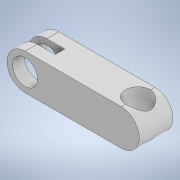
# Autodesk Inventor part: toplegV2
Saved by Autodesk Inventor 2022 (Build 260153000, 153)
## iProperties
Created: 2022-01-24
Part Number: toplegV2
Material: Generic
Document SubType Name: Modeling
Designer: money
Density: 1 g/cm^3
Appearance: Default
Author: money
Autodesk Inventor part; units mm, degrees
ref_plane "YZ Plane" through (0, 0, 0) normal (1, 0, 0) x (0, 1, 0)
ref_plane "XZ Plane" through (0, 0, 0) normal (0, 1, 0) x (-1, 0, 0)
ref_plane "XY Plane" through (0, 0, 0) normal (0, 0, 1) x (1, 0, 0)
sketch "Sketch1" plane through (0, 0, 0) normal (0, 0, 1) x (1, 0, 0)
  circle A0 centre (0, 0) radius 6.604
  arc A1 (0, 9.525) -> (0, -9.525) centre (0, 0) ccw
  line L0 (0, 9.525) -> (50.8, 9.525)
  line L1 (0, -9.525) -> (50.8, -9.525)
  arc A2 (50.8, -9.525) -> (50.8, 9.525) centre (50.8, 0) ccw
  dimension "d0" = 13.208
  dimension "d1" = 19.05
  dimension "d2" = 50.8
  dimension "d3" = 50.8
  dimension "d4" = 19.05
  constraints: 4 end point, 4 point on circle, 3 centre point, 2 coincident, 2 horizontal, 2 tangent
  measures "d0" diameter of A0
  measures "d1" diameter of A1
  measures "d2" distance of L1.start L1.end
  measures "d3" distance of L0.start L0.end
  measures "d4" diameter of A2
extrude "Extrusion1" add sketch "Sketch1" along normal blind 17.78
sketch "Sketch2" plane through (0, 0, 0) normal (0, 1, 0) x (-1, 0, 0)
  line L0 (9.525, 17.78) -> (0, 17.78) projected
  line L1 (9.525, 17.78) -> (9.525, 0)
  line L2 (9.525, 0) -> (9.525, 17.78) projected
  line L3 (0, 0) -> (0, 17.78) projected
  line L4 (9.525, 8.89) -> (0, 8.89)
  line L5 (0, 8.89) -> (0, 6.35)
  line L6 (0, 6.35) -> (9.525, 6.35)
  line L7 (9.525, 6.35) -> (9.525, 8.89)
  line L8 (9.525, 8.89) -> (0, 8.89)
  line L9 (0, 8.89) -> (0, 11.43)
  line L10 (0, 11.43) -> (9.525, 11.43)
  line L11 (9.525, 11.43) -> (9.525, 8.89)
  line L12 (0, 6.35) -> (-10.1637, 6.35)
  line L13 (-10.1637, 6.35) -> (-10.1637, 11.43)
  line L14 (-10.1637, 11.43) -> (0, 11.43)
  line L15 (0, 11.43) -> (0, 6.35)
  line L16 (9.525, 11.43) -> (-9.525, 11.43)
  line L17 (-9.525, 11.43) -> (-9.525, 6.35)
  line L18 (-9.525, 6.35) -> (9.525, 6.35)
  line L19 (9.525, 6.35) -> (9.525, 11.43)
  dimension "d8" = 2.54
  dimension "d9" = 2.54
  dimension "d10" = 19.05
  constraints: 34 end point, 8 parallel, 4 horizontal, 4 perpendicular, 4 point on line, 1 midpoint
  measures "d8" distance between parallel lines of L4 L6
  measures "d9" distance between parallel lines of L10 L4
  measures "d10" distance between parallel lines of L1 L17
extrude "Extrusion2" cut sketch "Sketch2" along normal mid plane 25.7175 contours L1 L4 L3 L10 | L3 L12 L17 L14 | L1 L6 L3 L4
sketch "Sketch3" plane through (0, 0, 0) normal (0, 1, 0) x (-1, 0, 0)
  line L0 (-50.8, 0) -> (-50.8, 17.78) projected
  circle A0 centre (-50.8, 8.89) radius 6.604
  point P0 (0, 0)
  dimension "d13" = 13.208
  constraints: 1 centre point, 1 midpoint
  measures "d13" diameter of A0
extrude "Extrusion3" cut sketch "Sketch3" along normal mid plane 25.7175
body "Solid1"
